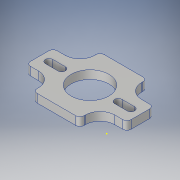
# Autodesk Inventor part: 4461-17-0101 Tensioner Plate
Saved by Autodesk Inventor 2018 (Build 220112000, 112)
## iProperties
Created: 2017-11-02
Part Number: 4461-17-0101 Tensioner Plate
Material: Aluminum 6061
Document SubType Name: Modeling
Designer: s-2513366
Density: 2.7 g/cm^3
Appearance: Aluminum - Flat
Mass: 50.8324 g
Surface Area: 84.0615 cm^2
Volume: 18.8268 cm^3
Author: s-2513366
Autodesk Inventor part; units mm, degrees
ref_plane "YZ Plane" through (0, 0, 0) normal (1, 0, 0) x (0, 1, 0)
ref_plane "XZ Plane" through (0, 0, 0) normal (0, 1, 0) x (-1, 0, 0)
ref_plane "XY Plane" through (0, 0, 0) normal (0, 0, 1) x (1, 0, 0)
sketch "Sketch1" plane through (0, 0, 0) normal (0, 1, 0) x (-1, 0, 0)
  line L0 (0, 0) -> (76.2, 0)
  line L1 (76.2, 0) -> (76.2, -50.8)
  line L2 (76.2, -50.8) -> (0, -50.8)
  line L3 (0, -50.8) -> (0, 0)
  dimension "d0" = 76.2
  dimension "d1" = 50.8
  constraints: 8 end point, 2 parallel, 1 horizontal, 1 perpendicular
  measures "d0" distance of L1.end L2.end
  measures "d1" distance of L0.end L1.end
extrude "Extrusion1" add sketch "Sketch1" along normal blind 6.35
sketch "Sketch2" plane through (0, 6.35, 0) normal (0, 1, 0) x (1, 0, 0)
  line L0 (0, 0) -> (0, 50.8) projected
  line L1 (-76.2, 50.8) -> (-76.2, 0) projected
  line L2 (0, 50.8) -> (-76.2, 0)
  line L3 (-76.2, 0) -> (-76.2, 50.8)
  line L4 (-76.2, 50.8) -> (0, 0)
  circle A0 centre (-38.1, 25.4) radius 14.2875
  dimension "d4" = 28.575
  constraints: 6 end point, 1 centre point, 1 collinear, 1 midpoint
  measures "d4" diameter of A0
hole "Hole1" at (-38.1, 6.35, -25.4) direction (0, -1, 0) diameter 28.575 end through all
sketch "Sketch3" plane through (0, 6.35, 0) normal (0, 1, 0) x (1, 0, 0)
  line L0 (0, 50.8) -> (0, 0) projected
  line L1 (0, 25.4) -> (-23.8125, 25.4)
  circle A0 centre (-38.1, 25.4) radius 14.2875 projected
  line L2 (-52.3875, 25.4) -> (-76.2, 25.4) construction
  line L3 (-76.2, 0) -> (-76.2, 50.8) projected
  line L4 (-69.0563, 25.4) -> (-59.5312, 25.4) construction
  line L5 (-69.0563, 22.606) -> (-59.5312, 22.606)
  line L6 (-59.5312, 28.194) -> (-69.0563, 28.194)
  arc A1 (-69.0563, 28.194) -> (-69.0563, 22.606) centre (-69.0563, 25.4) ccw
  arc A2 (-59.5312, 22.606) -> (-59.5312, 28.194) centre (-59.5312, 25.4) ccw
  line L7 (-16.6688, 25.4) -> (-7.1437, 25.4) construction
  line L8 (-16.6688, 22.606) -> (-7.1437, 22.606)
  line L9 (-7.1437, 28.194) -> (-16.6688, 28.194)
  arc A3 (-16.6688, 28.194) -> (-16.6688, 22.606) centre (-16.6688, 25.4) ccw
  arc A4 (-7.1437, 22.606) -> (-7.1437, 28.194) centre (-7.1437, 25.4) ccw
  point P0 (-64.2938, 25.4)
  point P1 (-11.9062, 25.4)
  dimension "d12" = 4.7625
  dimension "d13" = 5.588
  dimension "d14" = 4.7625
  dimension "d15" = 5.588
  constraints: 20 end point, 10 point on circle, 8 tangent, 6 midpoint, 4 centre point, 2 parallel, 2 point on line, 1 horizontal
  measures "d12" distance of point (-64.294, 25.4) L4.end
  measures "d13" diameter of A2
  measures "d14" distance of point (-11.906, 25.4) L7.end
  measures "d15" diameter of A4
extrude "Extrusion2" cut sketch "Sketch3" against normal blind 6.35 contours A4 L8 A3 L1 | L1 A3 L9 A4 | A1 L6 A2 L5
sketch "Sketch4" plane through (0, 6.35, 0) normal (0, 1, 0) x (1, 0, 0)
  point P0 (0, 0)
sketch "Sketch5" plane through (0, 6.35, 0) normal (0, 1, 0) x (1, 0, 0)
  line L0 (0, 0) -> (0, 50.8) projected
  line L1 (0, 0) -> (0, 15.24)
  line L2 (0, 15.24) -> (-20.32, 15.24)
  line L3 (-20.32, 15.24) -> (-20.32, 0)
  line L4 (0, 50.8) -> (-20.32, 50.8)
  line L5 (-20.32, 50.8) -> (-20.32, 35.56)
  line L6 (-20.32, 35.56) -> (0, 35.56)
  line L7 (0, 35.56) -> (0, 50.8)
  line L8 (0, 50.8) -> (-76.2, 50.8) projected
  line L9 (-76.2, 50.8) -> (-76.2, 35.56)
  line L10 (-76.2, 50.8) -> (-76.2, 0) projected
  line L11 (-76.2, 0) -> (0, 0) projected
  line L12 (-76.2, 0) -> (-76.2, 15.24)
  line L13 (-76.2, 15.24) -> (-55.88, 15.24)
  line L14 (-55.88, 15.24) -> (-55.88, 0)
  line L15 (-76.2, 35.56) -> (-55.88, 35.56)
  line L16 (-55.88, 35.56) -> (-55.88, 50.8)
  line L17 (-76.2, 0) -> (-55.88, 0)
  line L18 (-76.2, 15.24) -> (-55.88, 15.24)
  line L19 (-20.32, 0) -> (0, 0)
  line L20 (-55.88, 50.8) -> (-76.2, 50.8)
  dimension "d19" = 15.24
  dimension "d20" = 20.32
  dimension "d21" = 20.32
  dimension "d22" = 15.24
  dimension "d23" = 20.32
  constraints: 34 end point, 8 perpendicular, 4 point on line, 3 parallel, 2 horizontal, 1 collinear
  measures "d19" distance of L0.start L1.end
  measures "d20" distance of L1.end L2.end
  measures "d21" distance of L6.end L5.end
  measures "d22" distance of L4.end L5.end
  measures "d23" distance of L12.end L13.end
extrude "Extrusion3" cut sketch "Sketch5" against normal blind 25.4 contours L11 L3 L2 L0 | L6 L5 L4 L0 | L11 L10 L13 L14 | L16 L15 L9 L8
fillet "Fillet2" radius 3.175 8 edges at (-55.88, 3.175, -50.8) (-76.2, 3.175, -35.56) (-76.2, 3.175, -15.24) (-55.88, 3.175, 0) (0, 3.175, -15.24) (0, 3.175, -35.56) (-20.32, 3.175, -50.8) (-20.32, 3.175, 0)
fillet "Fillet3" radius 11.1125 4 edges at (-20.32, 3.175, -35.56) (-55.88, 3.175, -35.56) (-55.88, 3.175, -15.24) (-20.32, 3.175, -15.24)
body "Solid1"
